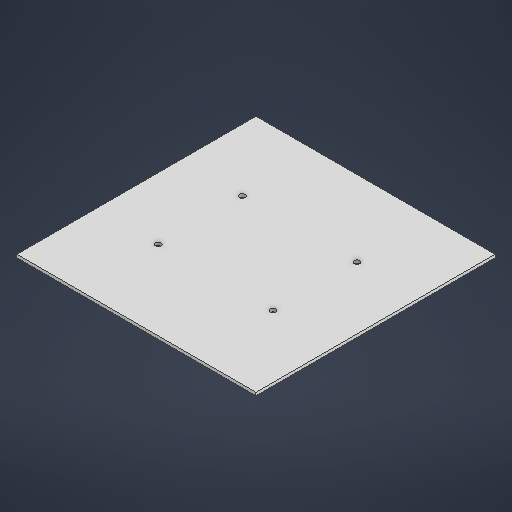
# Autodesk Inventor part: Pedalbox_V2_Floor
Saved by Autodesk Inventor 2026.1 (Build 301233000, 233)
## iProperties
Created: 2026-09-15
Part Number: Pedalbox_V2_Floor
Material: Generic
Document SubType Name: Modeling
Designer: share
Density: 1 g/cm^3
Appearance: Default
Author: share
Autodesk Inventor part; units mm, degrees
ref_plane "YZ Plane" through (0, 0, 0) normal (1, 0, 0) x (0, 1, 0)
ref_plane "XZ Plane" through (0, 0, 0) normal (0, 1, 0) x (-1, 0, 0)
ref_plane "XY Plane" through (0, 0, 0) normal (0, 0, 1) x (1, 0, 0)
sketch "Sketch1" plane through (0, 0, 0) normal (0, 1, 0) x (-1, 0, 0)
  line L0 (-125, 125) -> (125, 125)
  line L1 (125, 125) -> (125, -125)
  line L2 (125, -125) -> (-125, -125)
  line L3 (-125, -125) -> (-125, 125)
  line L4 (175, 0) -> (-175, 0) construction
  line L5 (0, -175) -> (0, 175) construction
  point P0 (0, 0)
  dimension "d0" = 250
  dimension "d1" = 250
  constraints: 8 end point, 2 parallel, 1 horizontal, 1 perpendicular, 2 other
  measures "d0" distance between parallel lines of L1 L3
  measures "d1" distance between parallel lines of L2 L0
extrude "Extrusion1" add sketch "Sketch1" along normal blind 3.175
sketch "Sketch2" plane through (0, 3.175, 0) normal (0, 1, 0) x (1, 0, 0)
  line L0 (0, 175) -> (0, -175) construction
  line L1 (175, 0) -> (-175, 0) construction
  line L2 (125, 125) -> (-125, 125) projected
  line L3 (60, -42.2089) -> (-60, -42.2089) construction
  line L4 (60, 45.5919) -> (-60, 45.5919) construction
  point P0 (0, 0)
  dimension "d4" = 79.4081
  dimension "d5" = 87.8008
  dimension "d6" = 120
  constraints: 4 end point, 2 horizontal, 2 symmetric about line, 1 parallel
  measures "d4" distance from line of L2 L4.start
  measures "d5" distance between parallel lines of L4 L3
  measures "d6" distance of L3.end L3.start
hole "Hole1" at (60, 3.175, -45.5919) at (-60, 3.175, -45.5919) at (60, 3.175, 42.2089) at (-60, 3.175, 42.2089) direction (0, -1, 0) diameter 6 end through all
body "Solid1"
